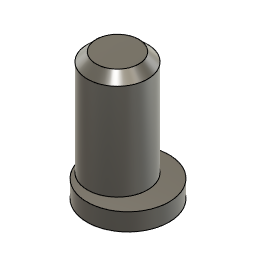
LuglessOpenSmartwatch_RoundButton v1 (Autodesk Fusion 360 design; units mm, degrees)
Autodesk Fusion 360 part; units mm, degrees
sketch "Sketch1" plane through (0, 0, 0) normal (1, 0, 0) x (0, 0, -1)
  circle A0 centre (0, 0) radius 21.5
  line L0 (19.85, -10.1) -> (-19.85, -10.1)
  line L1 (-19.85, -10.1) -> (-19.85, 10.1)
  line L2 (-19.85, 10.1) -> (19.85, 10.1)
  line L3 (19.85, 10.1) -> (19.85, -10.1)
  line L4 (19.85, -10.1) -> (-19.85, 10.1) construction
  line L5 (-19.85, -10.1) -> (19.85, 10.1) construction
  circle A1 centre (0, 0) radius 24
  line L6 (10.25, -26.5) -> (-10.25, -26.5)
  line L7 (-10.25, -26.5) -> (-10.25, 26.5)
  line L8 (-10.25, 26.5) -> (10.25, 26.5)
  line L9 (10.25, 26.5) -> (10.25, -26.5)
  line L10 (10.25, -26.5) -> (-10.25, 26.5) construction
  line L11 (-10.25, -26.5) -> (10.25, 26.5) construction
  line L12 (-10.25, 16.5) -> (10.25, 16.5)
  line L13 (-10.25, -16.5) -> (10.25, -16.5)
  dimension "CaseInnerDiameter" = 43
  dimension "BatteryLength" = 39.7
  dimension "BatteryWidth" = 20.2
  dimension "CaseWallThickness" = 2.5
  dimension "LugWidth" = 20.5
  dimension "StrapCutout" = 53
  dimension "UpperLugInset" = 10
  dimension "LowerLugInset" = 10
  constraint coincident A0.centre A1.centre
  constraint horizontal L0
  constraint perpendicular L0 L1
  constraint parallel L0 L2
  constraint parallel L1 L3
  constraint coincident L4 A0.centre
  constraint coincident L5 A0.centre
  constraint horizontal L6
  constraint perpendicular L6 L7
  constraint parallel L6 L8
  constraint parallel L7 L9
  constraint coincident L10 A0.centre
  constraint coincident L11 A0.centre
  constraint coincident L7 L12.start
  constraint coincident L9 L12.end
  constraint perpendicular L9 L12
  constraint coincident L7 L13.start
  constraint coincident L9 L13.end
  constraint perpendicular L9 L13
  measures "CaseInnerDiameter" diameter of A0
  measures "BatteryLength" distance of L1.end L2.end
  measures "BatteryWidth" distance of L0.end L1.end
  measures "CaseWallThickness" distance of A0 A1
  measures "LugWidth" distance of L7.end L8.end
  measures "StrapCutout" distance of L6.end L7.end
  measures "UpperLugInset" distance of L8 L12
  measures "LowerLugInset" distance of L6 L13
sketch "Sketch19" plane through (0, 0, 0) normal (0, 1, 0) x (1, 0, 0)
  circle A0 centre (-0.2453, 29.9832) radius 1.725
  circle A1 centre (0.3438, 29.9967) radius 2.35
  dimension "d142" = 3.45
  dimension "d145" = 4.7
  measures "d142" diameter of A0
  measures "d145" diameter of A1
extrude "Extrude28" add sketch "Sketch19" against normal blind 1 contours A0 | A1 makes body 1
extrude "Extrude27" add sketch "Sketch19" along normal blind 6 separate body contours A0 makes body 2
combine "Combine3" operation add target body 1 tool bodies 2
chamfer "Chamfer9" distance 0.5 angle 45 1 edges at (-1.8536, 6, -29.3595) on bodies 1
equation "StrapCutout = CaseInnerDiameter + 10 mm"
equation "BottomCaseLipChamfer = 1.20 mm"
equation "UpperCaseThickness = 5.77 mm"
